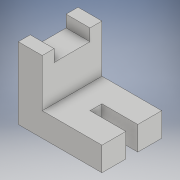
# Autodesk Inventor part: 4.1e P3
Saved by Autodesk Inventor 2017.1 (Build 211199000, 199)
## iProperties
Created: 2016-10-22
Part Number: 4.1e P3
Material: Generic
Document SubType Name: Modeling
Designer: rbibby53
Density: 1 g/cm^3
Appearance: Default
Author: rbibby53
Autodesk Inventor part; units mm, degrees
ref_plane "YZ Plane" through (0, 0, 0) normal (1, 0, 0) x (0, 1, 0)
ref_plane "XZ Plane" through (0, 0, 0) normal (0, 1, 0) x (-1, 0, 0)
ref_plane "XY Plane" through (0, 0, 0) normal (0, 0, 1) x (1, 0, 0)
sketch "Sketch1" plane through (0, 0, 0) normal (1, 0, 0) x (0, 1, 0)
  line L0 (10.6243, 20.9647) -> (-52.8757, 20.9647)
  line L1 (-52.8757, 20.9647) -> (-52.8757, -42.5353)
  line L2 (-52.8757, -42.5353) -> (10.6243, -42.5353)
  line L3 (10.6243, -42.5353) -> (10.6243, 20.9647)
  point P0 (0, 0)
  dimension "d0" = 63.5
  dimension "d1" = 63.5
  constraints: 8 end point, 2 parallel, 1 horizontal, 1 perpendicular
  measures "d0" distance of L2.end L1.end
  measures "d1" distance of L1.end L0.end
extrude "Extrusion1" add sketch "Sketch1" along normal blind 25.4
sketch "Sketch2" plane through (25.4, 0, 0) normal (1, 0, 0) x (0, 0, -1)
  line L0 (42.5353, 10.6243) -> (-20.9647, 10.6243) projected
  line L1 (-20.9647, 10.6243) -> (-8.2647, 10.6243)
  line L2 (-8.2647, 10.6243) -> (-8.2647, 23.3243)
  line L3 (-8.2647, 23.3243) -> (-20.9647, 23.3243)
  line L4 (-20.9647, 23.3243) -> (-20.9647, 10.6243)
  line L5 (42.5353, -52.8757) -> (42.5353, 10.6243) projected
  line L6 (42.5353, 10.6243) -> (29.8353, 10.6243)
  line L7 (29.8353, 10.6243) -> (29.8353, 23.3243)
  line L8 (29.8353, 23.3243) -> (42.5353, 23.3243)
  line L9 (42.5353, 23.3243) -> (42.5353, 10.6243)
  point P0 (0, 0)
  dimension "d4" = 12.7
  dimension "d5" = 12.7
  dimension "d6" = 12.7
  dimension "d7" = 12.7
  constraints: 16 end point, 4 parallel, 2 horizontal, 2 perpendicular
  measures "d4" distance of L3.end L2.end
  measures "d5" distance of L2.end L1.end
  measures "d6" distance of L7.end L8.end
  measures "d7" distance of L6.end L7.end
extrude "Extrusion2" add sketch "Sketch2" against normal blind 25.4
sketch "Sketch3" plane through (25.4, 0, 0) normal (1, 0, 0) x (0, 0, -1)
  line L0 (-20.9647, -52.8757) -> (42.5353, -52.8757)
  line L1 (42.5353, -52.8757) -> (42.5353, -27.4757)
  line L2 (42.5353, -27.4757) -> (-20.9647, -27.4757)
  line L3 (-20.9647, -27.4757) -> (-20.9647, -52.8757)
  point P0 (0, 0)
  dimension "d10" = 63.5
  dimension "d11" = 25.4
  constraints: 8 end point, 2 parallel, 1 horizontal, 1 perpendicular
  measures "d10" distance of L2.end L1.end
  measures "d11" distance of L1.end L0.end
extrude "Extrusion3" add sketch "Sketch3" along normal blind 63.5
sketch "Sketch4" plane through (88.9, 0, 0) normal (1, 0, 0) x (0, 0, -1)
  line L0 (-20.9647, 23.3243) -> (-20.9647, -52.8757) projected
  line L1 (-20.9647, -52.8757) -> (4.4353, -52.8757)
  line L2 (-20.9647, -52.8757) -> (42.5353, -52.8757) projected
  line L3 (4.4353, -52.8757) -> (4.4353, -27.4757)
  line L4 (42.5353, -27.4757) -> (-20.9647, -27.4757) projected
  line L5 (42.5353, -52.8757) -> (42.5353, -27.4757) projected
  line L6 (42.5353, -52.8757) -> (17.1353, -52.8757)
  line L7 (17.1353, -52.8757) -> (17.1353, -27.4757)
  line L8 (4.4353, -27.4757) -> (17.1353, -27.4757)
  line L9 (17.1353, -27.4757) -> (17.1353, -52.8757)
  line L10 (17.1353, -52.8757) -> (4.4353, -52.8757)
  line L11 (4.4353, -52.8757) -> (4.4353, -27.4757)
  point P0 (0, 0)
  dimension "d14" = 25.4
  dimension "d15" = 25.4
  constraints: 16 end point, 3 perpendicular, 3 point on line, 2 parallel, 1 horizontal
  measures "d14" distance of L0.end L1.end
  measures "d15" distance of L2.end L6.end
extrude "Extrusion4" cut sketch "Sketch4" against normal blind 38.1 contours L4 L7 L2 L3
body "Solid1"
